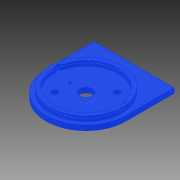
# Autodesk Inventor part: WhitePumpBase
Saved by Autodesk Inventor 2013 (Build 170138000, 138)
## iProperties
Created: 2014-07-16
Part Number: WhitePumpBase
Material: Generic
Document SubType Name: Modeling
Designer: Dan
Density: 1 g/cm^3
Author: Dan
Autodesk Inventor part; units mm, degrees
ref_plane "YZ Plane" through (0, 0, 0) normal (1, 0, 0) x (0, 1, 0)
ref_plane "XZ Plane" through (0, 0, 0) normal (0, 1, 0) x (-1, 0, 0)
ref_plane "XY Plane" through (0, 0, 0) normal (0, 0, 1) x (1, 0, 0)
sketch "Sketch1" plane through (0, 0, 0) normal (0, 1, 0) x (-1, 0, 0)
  arc A0 (20, 0) -> (-20, 0) centre (0, 0) ccw
  line L0 (20, 0) -> (20, -24)
  line L1 (20, -24) -> (-20, -24)
  line L2 (-20, -24) -> (-20, 0)
  dimension "d0" = 40
  dimension "d1" = 44
  constraints: 6 end point, 2 point on circle, 2 tangent, 1 centre point, 1 coincident, 1 horizontal, 1 parallel, 1 vertical
  measures "d0" diameter of A0
extrude "Extrusion1" add sketch "Sketch1" along normal blind 2.5
sketch "Sketch2" plane through (0, 2.5, 0) normal (0, 1, 0) x (1, 0, 0)
  arc A0 (-20, 0) -> (20, 0) centre (0, 0) ccw projected
  circle A1 centre (0, 0) radius 18
  circle A2 centre (0, 0) radius 16
  arc A3 (-15.6171, 3.4796) -> (-15.9875, 0.6328) centre (-15.3704, 2) ccw
  arc A4 (15.9875, 0.6328) -> (15.6171, 3.4796) centre (15.3704, 2) ccw
  line L0 (-15.8662, 2.0645) -> (-16.8579, 2.1935) construction
  line L1 (16.8579, 2.1935) -> (15.8662, 2.0645) construction
  dimension "d4" = 36
  dimension "d7" = 2
  dimension "d8" = 3
  dimension "d9" = 1
  dimension "d10" = 2
  constraints: 12 point on circle, 4 centre point, 4 end point, 4 line through centre, 2 coincident, 1 equal length, 1 equal radius, 1 horizontal alignment
  measures "d4" diameter of A1
  measures "d7" radial gap between concentric circles of A1 A2
  measures "d8" diameter of A3
  measures "d9" distance of L0.start L0.end
  measures "d10" vertical distance of A0.centre A3.centre
extrude "Extrusion2" add sketch "Sketch2" along normal blind 2.5
sketch "Sketch3" plane through (0, 2.5, 0) normal (0, 1, 0) x (1, 0, 0)
  arc A0 (-15.9875, 0.6328) -> (15.9875, 0.6328) centre (0, 0) ccw projected
  circle A1 centre (0, 0) radius 3.125
  dimension "d13" = 6.25
  constraints: 1 centre point, 1 coincident
  measures "d13" diameter of A1
extrude "Extrusion3" cut sketch "Sketch3" against normal through all
sketch "Sketch4" plane through (0, 2.5, 0) normal (0, 1, 0) x (1, 0, 0)
  circle A0 centre (0, 0) radius 3.125 projected
  circle A1 centre (-8, 0) radius 0.625
  dimension "d16" = 1.25
  dimension "d18" = 8
  constraints: 1 centre point
  measures "d16" diameter of A1
  measures "d18" distance of A1.centre A0.centre
extrude "Extrusion4" add sketch "Sketch4" along normal blind 1 contours A1
sketch "Sketch5" plane through (0, 2.5, 0) normal (0, 1, 0) x (1, 0, 0)
  circle A0 centre (0, 0) radius 3.125 projected
  circle A1 centre (7.7782, 7.7782) radius 1.435
  circle A2 centre (-7.7782, -7.7782) radius 1.435
  line L0 (7.7782, 7.7782) -> (-7.7782, -7.7782) construction
  line L1 (20, 24) -> (-20, 24) construction
  dimension "d21" = 2.87
  dimension "d23" = 22
  dimension "d24" = 45
  constraints: 2 centre point, 2 end point, 1 coincident, 1 equal radius, 1 midpoint
  measures "d21" diameter of A2
  measures "d23" distance of L0.start L0.end
  measures "d24" angle of L1 L0
extrude "Extrusion5" cut sketch "Sketch5" against normal through all contours A1 | A2
body "Solid1"
